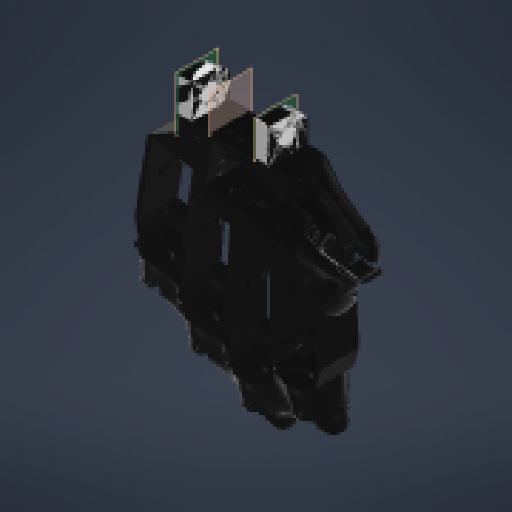
# Autodesk Inventor part: i2_WristLargeV2
Saved by Autodesk Inventor 2024 (Build 280153000, 153)
## iProperties
Created: 2025-09-27
Part Number: i2_WristLargeV2
Material: Generic
Document SubType Name: Modeling
Designer: kevin
Density: 1 g/cm^3
Appearance: Default
Author: kevin
Autodesk Inventor part; units mm, degrees
ref_plane "YZ Plane" through (0, 0, 0) normal (1, 0, 0) x (0, 1, 0)
ref_plane "XZ Plane" through (0, 0, 0) normal (0, 1, 0) x (-1, 0, 0)
ref_plane "XY Plane" through (0, 0, 0) normal (0, 0, 1) x (1, 0, 0)
sketch "Sketch2" plane through (9.6191, 85.8932, 0) normal (1, 0, 0) x (0, 1, 0)
  line L0 (5.8475, 19.7393) -> (-11.4347, 19.7393) projected
  line L1 (-11.4347, 19.7393) -> (-11.4376, 0.0015) projected
  line L2 (-11.4365, 0.0015) -> (0, -0.0006) projected
  line L3 (0, 0) -> (1.7975, 1.364) projected
  circle A0 centre (-3.2032, 8.8788) radius 9.0266 projected
  line L4 (5.6735, 7.164) -> (5.8475, 19.7393) projected
  point P0 (-85.8932, 0)
  point P1 (5.6747, 7.2472)
  point P2 (-11.4368, 5.179)
  point P3 (-4.8319, 0.0003)
  point P4 (-1.5779, -0.0003)
  constraints: 1 other
sketch "Sketch3" plane through (-29.9469, 82.6227, 0) normal (1, 0, 0) x (0, 1, 0)
  line L0 (9.1181, 19.7392) -> (-8.1642, 19.7392) projected
  line L1 (-8.1642, 19.7392) -> (-8.1663, 5.179) projected
  arc A0 (-8.1663, 5.179) -> (-1.5614, 0.0002) centre (0.0673, 8.8787) ccw projected
  line L2 (-1.5614, 0.0002) -> (1.6926, -0.0004) projected
  arc A1 (1.6926, -0.0004) -> (8.9452, 7.2471) centre (0.0673, 8.8787) ccw projected
  line L3 (8.9452, 7.2471) -> (9.1181, 19.7392) projected
  point P0 (-82.6227, 0)
ref_plane "Work Plane1" through (-36.8289, 82.6227, 19.7393) normal (-1, -0.0002, 0.0001) x (0.0002, -1, 0)
ref_plane "Work Plane2" through (2.7431, 81.7427, 6.6) normal (-1, 0, 0) x (0, -1, 0)
extrude "Extrusion3" add sketch "Sketch2" against normal up to surface (6.876 mm away) contours L4 A0 L1 L0 | L4 A0 L2 L1
extrude "Extrusion4" add sketch "Sketch3" against normal up to surface (6.8837 mm away)
ref_plane "Work Plane3" through (-19.9469, 82.6227, 0) normal (1, 0, 0) x (0, 0, -1)
body "Solid2"
